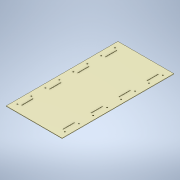
# Autodesk Inventor part: top_bottom_layer_3mm
Saved by Autodesk Inventor 2021 (Build 250183000, 183)
## iProperties
Created: 2021-01-27
Part Number: top_bottom_layer_3mm
Material: Acrylic
Document SubType Name: Modeling
Designer: abij996
Density: 1.188 g/cm^3
Appearance: Smooth - Ash
Author: abij996
Autodesk Inventor part; units mm, degrees
ref_plane "YZ Plane" through (0, 0, 0) normal (1, 0, 0) x (0, 1, 0)
ref_plane "XZ Plane" through (0, 0, 0) normal (0, 1, 0) x (-1, 0, 0)
ref_plane "XY Plane" through (0, 0, 0) normal (0, 0, 1) x (1, 0, 0)
sketch "Sketch2" plane through (0, 0, 0) normal (0, 1, 0) x (-1, 0, 0)
  line L0 (238.7833, 367.5648) -> (-161.2167, 367.5648)
  line L1 (-161.2167, 367.5648) -> (-161.2167, -432.4352)
  line L2 (-161.2167, -432.4352) -> (238.7833, -432.4352)
  line L3 (238.7833, -432.4352) -> (238.7833, 367.5648)
  circle A0 centre (208.7833, 217.5648) radius 4
  circle A1 centre (208.7833, 317.5648) radius 4
  circle A2 centre (209.7833, -382.4352) radius 4
  circle A3 centre (209.7833, -283.981) radius 4
  circle A4 centre (209.7833, -183.981) radius 4
  circle A5 centre (209.7833, -83.981) radius 4
  circle A6 centre (209.7833, 16.019) radius 4
  circle A7 centre (209.7833, 116.019) radius 4
  line L4 (38.7833, -432.4352) -> (38.7833, 367.5648) construction
  circle A8 centre (-131.2167, 217.5648) radius 4
  circle A9 centre (-131.2167, 317.5648) radius 4
  circle A10 centre (-132.2167, -382.4352) radius 4
  circle A11 centre (-132.2167, -283.981) radius 4
  circle A12 centre (-132.2167, -183.981) radius 4
  circle A13 centre (-132.2167, -83.981) radius 4
  circle A14 centre (-132.2167, 16.019) radius 4
  circle A15 centre (-132.2167, 116.019) radius 4
  line L5 (188.7833, -372.4352) -> (185.2833, -372.4352)
  line L6 (185.2833, -372.4352) -> (185.2833, -292.4352)
  line L7 (185.2833, -292.4352) -> (188.7833, -292.4352)
  line L8 (188.7833, -292.4352) -> (188.7833, -372.4352)
  line L9 (188.7833, -172.4352) -> (185.2833, -172.4352)
  line L10 (185.2833, -172.4352) -> (185.2833, -92.4352)
  line L11 (185.2833, -92.4352) -> (188.7833, -92.4352)
  line L12 (188.7833, -92.4352) -> (188.7833, -172.4352)
  line L13 (188.7833, 27.5648) -> (185.2833, 27.5648)
  line L14 (185.2833, 27.5648) -> (185.2833, 107.5648)
  line L15 (185.2833, 107.5648) -> (188.7833, 107.5648)
  line L16 (188.7833, 107.5648) -> (188.7833, 27.5648)
  line L17 (188.7833, 227.5648) -> (185.2833, 227.5648)
  line L18 (185.2833, 227.5648) -> (185.2833, 307.5648)
  line L19 (185.2833, 307.5648) -> (188.7833, 307.5648)
  line L20 (188.7833, 307.5648) -> (188.7833, 227.5648)
  line L21 (-111.2167, -372.4352) -> (-107.7167, -372.4352)
  line L22 (-107.7167, -372.4352) -> (-107.7167, -292.4352)
  line L23 (-107.7167, -292.4352) -> (-111.2167, -292.4352)
  line L24 (-111.2167, -292.4352) -> (-111.2167, -372.4352)
  line L25 (-111.2167, -172.4352) -> (-107.7167, -172.4352)
  line L26 (-107.7167, -172.4352) -> (-107.7167, -92.4352)
  line L27 (-107.7167, -92.4352) -> (-111.2167, -92.4352)
  line L28 (-111.2167, -92.4352) -> (-111.2167, -172.4352)
  line L29 (-111.2167, 27.5648) -> (-107.7167, 27.5648)
  line L30 (-107.7167, 27.5648) -> (-107.7167, 107.5648)
  line L31 (-107.7167, 107.5648) -> (-111.2167, 107.5648)
  line L32 (-111.2167, 107.5648) -> (-111.2167, 27.5648)
  line L33 (-111.2167, 227.5648) -> (-107.7167, 227.5648)
  line L34 (-107.7167, 227.5648) -> (-107.7167, 307.5648)
  line L35 (-107.7167, 307.5648) -> (-111.2167, 307.5648)
  line L36 (-111.2167, 307.5648) -> (-111.2167, 227.5648)
  point P0 (0, 0)
  dimension "d46" = 800
  dimension "d47" = 400
  dimension "d51" = 8
  dimension "d52" = 30
  dimension "d53" = 650
  dimension "d58" = 8
  dimension "d60" = 30
  dimension "d61" = 50
  dimension "d66" = 8
  dimension "d67" = 50
  dimension "d68" = 8
  dimension "d69" = 8
  dimension "d70" = 8
  dimension "d71" = 8
  dimension "d72" = 8
  dimension "d73" = 3.5
  dimension "d74" = 80
  dimension "d75" = 80
  dimension "d76" = 80
  dimension "d77" = 80
  dimension "d78" = 3.5
  dimension "d79" = 3.5
  dimension "d80" = 3.5
  dimension "d81" = 50
  dimension "d82" = 50
  dimension "d83" = 60
  dimension "d84" = 120
  dimension "d85" = 120
  dimension "d86" = 120
  constraints: 74 end point, 24 symmetric about line, 16 centre point, 10 parallel, 5 horizontal, 5 perpendicular, 4 point on line, 2 midpoint, 8 other
  measures "d46" distance of L2.end L0.start
  measures "d47" distance of L0.start L0.end
  measures "d51" diameter of A0
  measures "d52" distance from line of L3 A0.centre
  measures "d53" distance from line of L2 A0.centre
  measures "d58" diameter of A1
  measures "d60" distance from line of L3 A1.centre
  measures "d61" distance from line of L0 A1.centre
  measures "d66" diameter of A2
  measures "d67" distance from line of L2 A2.centre
  measures "d68" diameter of A3
  measures "d69" diameter of A4
  measures "d70" diameter of A5
  measures "d71" diameter of A6
  measures "d72" diameter of A7
  measures "d73" distance between parallel lines of L6 L8
  measures "d74" distance of L5.end L6.end
  measures "d75" distance of L9.end L10.end
  measures "d76" distance of L13.end L14.end
  measures "d77" distance of L17.end L18.end
  measures "d78" distance of L14.end L15.end
  measures "d79" distance of L17.start L17.end
  measures "d80" distance of L9.start L9.end
  measures "d81" distance between parallel lines of L3 L8
  measures "d82" distance between parallel lines of L3 L12
  measures "d83" distance between parallel lines of L0 L19
  measures "d84" distance between parallel lines of L15 L17
  measures "d85" distance between parallel lines of L11 L13
  measures "d86" distance between parallel lines of L7 L9
extrude "Extrusion6" add sketch "Sketch2" along normal blind 3
body "Solid6"
